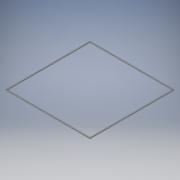
# Autodesk Inventor part: Rahmen
Saved by Autodesk Inventor 2019 (Build 230136000, 136)
## iProperties
Created: 2021-09-27
Part Number: Rahmen
Material: Generisch
Document SubType Name: Modeling
Designer: mritt
Density: 1 g/cm^3
Appearance: Vorgabe
Mass: 1813.5 g
Surface Area: 4836 cm^2
Volume: 1813.5 cm^3
Author: mritt
Autodesk Inventor part; units mm, degrees
ref_plane "YZ Plane" through (0, 0, 0) normal (1, 0, 0) x (0, 1, 0)
ref_plane "XZ Plane" through (0, 0, 0) normal (0, 1, 0) x (-1, 0, 0)
ref_plane "XY Plane" through (0, 0, 0) normal (0, 0, 1) x (1, 0, 0)
sketch "Skizze1" plane through (0, 0, 0) normal (0, 1, 0) x (-1, 0, 0)
  line L0 (2324.7965, -1368.0982) -> (324.7965, -1368.0982)
  line L1 (324.7965, -1368.0982) -> (324.7965, -3368.0982)
  line L2 (324.7965, -3368.0982) -> (2324.7965, -3368.0982)
  line L3 (2324.7965, -3368.0982) -> (2324.7965, -1368.0982)
  line L4 (309.7965, -1353.0982) -> (2339.7965, -1353.0982)
  line L5 (2339.7965, -1353.0982) -> (2339.7965, -3383.0982)
  line L6 (2339.7965, -3383.0982) -> (309.7965, -3383.0982)
  line L7 (309.7965, -3383.0982) -> (309.7965, -1353.0982)
  line L8 (309.7965, -1353.0982) -> (2339.7965, -3383.0982) construction
  line L9 (2339.7965, -1353.0982) -> (309.7965, -3383.0982) construction
  point P0 (0, 0)
  point P1 (1324.7965, -2368.0982)
  dimension "d0" = 2000
  dimension "d1" = 2000
  dimension "d2" = 15
  dimension "d3" = 15
  dimension "d4" = 15
  dimension "d5" = 15
  constraints: 20 end point, 4 parallel, 2 horizontal, 2 midpoint, 2 perpendicular
  measures "d0" distance of L0.end L1.end
  measures "d1" distance of L1.end L2.end
  measures "d2" distance between parallel lines of L3 L5
  measures "d3" distance between parallel lines of L4 L0
  measures "d4" distance between parallel lines of L1 L7
  measures "d5" distance between parallel lines of L2 L6
extrude "Extrusion1" add sketch "Skizze1" along normal blind 15
